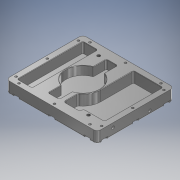
# Autodesk Inventor part: bottom plate mod
Saved by Autodesk Inventor 2017 SP1 (Build 210196100, 196)
## iProperties
Created: 2018-05-03
Part Number: bottom plate mod
Material: Aluminum 6061
Document SubType Name: Modeling
Designer: SimonD
Density: 2.7 g/cm^3
Appearance: Aluminum - Polished
Author: SimonD
Autodesk Inventor part; units mm, degrees
ref_plane "YZ Plane" through (0, 0, 0) normal (1, 0, 0) x (0, 1, 0)
ref_plane "XZ Plane" through (0, 0, 0) normal (0, 1, 0) x (-1, 0, 0)
ref_plane "XY Plane" through (0, 0, 0) normal (0, 0, 1) x (1, 0, 0)
sketch "Sketch1" plane through (0, 0, 0) normal (0, 0, 1) x (1, 0, 0)
  line L0 (-53, 53) -> (53, 53)
  line L1 (53, 53) -> (53, -53)
  line L2 (53, -53) -> (-53, -53)
  line L3 (-53, -53) -> (-53, 53)
  line L4 (-53, 53) -> (53, -53) construction
  line L5 (53, 53) -> (-53, -53) construction
  point P0 (0, 0)
  dimension "d0" = 106
  dimension "d1" = 106
  constraints: 12 end point, 2 midpoint, 2 parallel, 1 horizontal, 1 perpendicular
  measures "d0" distance of L1.end L2.end
  measures "d1" distance between parallel lines of L2 L0
extrude "Extrusion1" add sketch "Sketch1" along normal blind 16
sketch "Sketch3" plane through (0, 0, 16) normal (0, 0, 1) x (1, 0, 0)
  circle A0 centre (0, 0) radius 23.25
  dimension "d21" = 46.5
  constraints: 1 centre point, 1 coincident
  measures "d21" diameter of A0
extrude "Extrusion2" cut sketch "Sketch3" against normal blind 12
thicken "Thicken1" operation add thickness 20 both sides no extend neighbours yes toward (1, 0, 0) faces at (53, 17.6667, 5.3333)
fillet "Fillet3" radius 5 4 edges at (-53, -53, 8) (-53, 53, 8) (73, -53, 8) (73, 53, 8)
sketch "Sketch4" plane through (0, 0, 0) normal (0, 0, -1) x (-1, 0, 0)
  line L0 (48, 53) -> (-68, 53) projected
  line L1 (-73, 48) -> (-73, -48) projected
  line L2 (53, -48) -> (53, 48) projected
  line L3 (-68, -53) -> (48, -53) projected
  point P0 (0, 0)
  point P1 (-59, 49)
  point P2 (-69, 0)
  point P3 (-59, -49)
  point P4 (-10, -49)
  point P5 (39, -49)
  point P6 (49, 0)
  point P7 (39, 49)
  point P8 (-10, 49)
  point P9 (49, 43)
  point P10 (49, -43)
  point P11 (-69, 43)
  point P12 (-69, -43)
  dimension "d28" = 4
  dimension "d29" = 14
  dimension "d30" = 14
  dimension "d31" = 4
  dimension "d32" = 4
  dimension "d33" = 4
  dimension "d34" = 14
  dimension "d35" = 4
  dimension "d36" = 14
  dimension "d37" = 4
  dimension "d38" = 4
  dimension "d39" = 63
  dimension "d40" = 63
  dimension "d43" = 10
  dimension "d44" = 10
  dimension "d45" = 4
  dimension "d53" = 4
  measures "d28" distance from line of point (-59, 49) L0
  measures "d29" distance from line of point (-59, 49) L1
  measures "d30" distance from line of point (39, 49) L2
  measures "d31" distance from line of point (-10, 49) L0
  measures "d32" distance from line of point (-69, 0) L1
  measures "d33" distance from line of point (-59, -49) L3
  measures "d34" distance from line of point (-59, -49) L1
  measures "d35" distance from line of point (39, -49) L3
  measures "d36" distance from line of point (39, -49) L2
  measures "d37" distance from line of point (-10, -49) L3
  measures "d38" distance from line of point (49, 0) L2
  measures "d39" distance from line of point (-10, 49) L1
  measures "d40" distance from line of point (-10, -49) L1
  measures "d43" distance from line of point (49, 43) L0
  measures "d44" distance from line of point (49, -43) L3
  measures "d45" distance from line of point (49, -43) L2
  measures "d53" distance from line of point (39, 49) L0
hole "Hole2" at (59, 49, 0) at (69, 0, 0) at (59, -49, 0) at (10, -49, 0) at (-39, -49, 0) at (-49, 0, 0) at (-39, 49, 0) at (10, 49, 0) at (-49, 43, 0) at (-49, -43, 0) at (69, -43, 0) at (69, 43, 0) direction (0, 0, 1) diameter 3.1 end through all
fillet "Fillet5" radius 2 8 edges at (71.5355, 51.5355, 0) (73, 0, 0) (71.5355, -51.5355, 0) (10, -53, 0) (-51.5355, -51.5355, 0) (-53, 0, 0) (-51.5355, 51.5355, 0) (10, 53, 0)
sketch "Sketch7" plane through (0, 0, 16) normal (0, 0, 1) x (1, 0, 0)
  line L0 (7.5, -40) -> (-7.5, -40)
  line L1 (-7.5, -40) -> (-7.5, 40)
  line L2 (-7.5, 40) -> (7.5, 40)
  line L3 (7.5, 40) -> (7.5, -40)
  line L4 (7.5, -40) -> (-7.5, 40) construction
  line L5 (-7.5, -40) -> (7.5, 40) construction
  point P0 (0, 0)
  dimension "d78" = 15
  dimension "d157" = 40
  constraints: 12 end point, 2 midpoint, 2 parallel, 1 horizontal, 1 perpendicular
  measures "d78" distance of L1.end L2.end
  measures "d157" distance from line of L2 point (0, 0)
extrude "Extrusion4" cut sketch "Sketch7" against normal blind 12
fillet "Fillet6" radius 2 4 edges at (-7.5, 40, 10) (7.5, 40, 10) (-7.5, -40, 10) (7.5, -40, 10)
chamfer "Chamfer1" distance 0.5 angle 45 16 edges at (6.9142, -39.4142, 16) (7.5, -30.0036, 16) (0, -40, 16) (-6.9142, -39.4142, 16) (-7.5, -30.0036, 16) (-23.25, 0, 16) (-7.5, 30.0036, 16) (-6.9142, 39.4142, 16) (0, 40, 16) (6.9142, 39.4142, 16) (7.5, 30.0036, 16) (-7.5, 22.0071, 10) (7.5, 22.0071, 10) (-7.5, -22.0071, 10) (7.5, -22.0071, 10) (23.25, 0, 16)
sketch "Sketch8" plane through (0, 0, 0) normal (0, 0, -1) x (-1, 0, 0)
  circle A0 centre (39, -49) radius 1.55 projected
  circle A1 centre (49, -43) radius 1.55 projected
  circle A2 centre (49, 0) radius 1.55 projected
  circle A3 centre (-59, -49) radius 1.55 projected
  circle A4 centre (-69, 0) radius 1.55 projected
  circle A5 centre (-59, 49) radius 1.55 projected
  circle A6 centre (-10, 49) radius 1.55 projected
  circle A7 centre (39, 49) radius 1.55 projected
  circle A8 centre (49, 43) radius 1.55 projected
  line L0 (53, -3) -> (46, -3)
  line L1 (46, -3) -> (46, 3)
  line L2 (46, 3) -> (53, 3)
  line L3 (53, 3) -> (53, -3)
  line L4 (53, -48) -> (53, 48) projected
  line L5 (53, 40) -> (46, 40)
  line L6 (46, 40) -> (46, 46)
  line L7 (46, 46) -> (53, 46)
  line L8 (53, 46) -> (53, 40)
  line L9 (48, 53) -> (-68, 53) projected
  line L10 (42, 46) -> (36, 46)
  line L11 (36, 46) -> (36, 53)
  line L12 (36, 53) -> (42, 53)
  line L13 (42, 53) -> (42, 46)
  line L14 (-7, 46) -> (-13, 46)
  line L15 (-13, 46) -> (-13, 53)
  line L16 (-13, 53) -> (-7, 53)
  line L17 (-7, 53) -> (-7, 46)
  line L18 (-56, 46) -> (-62, 46)
  line L19 (-62, 46) -> (-62, 53)
  line L20 (-62, 53) -> (-56, 53)
  line L21 (-56, 53) -> (-56, 46)
  line L22 (-73, -3) -> (-66, -3)
  line L23 (-66, -3) -> (-66, 3)
  line L24 (-66, 3) -> (-73, 3)
  line L25 (-73, 3) -> (-73, -3)
  line L26 (-56, -53) -> (-62, -53)
  line L27 (-62, -53) -> (-62, -46)
  line L28 (-62, -46) -> (-56, -46)
  line L29 (-56, -46) -> (-56, -53)
  line L30 (42, -53) -> (36, -53)
  line L31 (36, -53) -> (36, -46)
  line L32 (36, -46) -> (42, -46)
  line L33 (42, -46) -> (42, -53)
  line L34 (53, -46) -> (46, -46)
  line L35 (46, -46) -> (46, -40)
  line L36 (46, -40) -> (53, -40)
  line L37 (53, -40) -> (53, -46)
  line L38 (-7, -53) -> (-13, -53)
  line L39 (-13, -53) -> (-13, -46)
  line L40 (-13, -46) -> (-7, -46)
  line L41 (-7, -46) -> (-7, -53)
  circle A9 centre (-10, -49) radius 1.55 projected
  line L42 (-73, 48) -> (-73, -48) projected
  line L43 (-73, 40) -> (-66, 40)
  line L44 (-66, 40) -> (-66, 46)
  line L45 (-66, 46) -> (-73, 46)
  line L46 (-73, 46) -> (-73, 40)
  line L47 (-73, -46) -> (-66, -46)
  line L48 (-66, -46) -> (-66, -40)
  line L49 (-66, -40) -> (-73, -40)
  line L50 (-73, -40) -> (-73, -46)
  circle A10 centre (-69, -43) radius 1.55 projected
  circle A11 centre (-69, 43) radius 1.55 projected
  point P0 (0, 0)
  point P1 (-7, -53)
  dimension "d85" = 3
  dimension "d86" = 3
  dimension "d87" = 3
  dimension "d88" = 3
  dimension "d89" = 3
  dimension "d90" = 3
  dimension "d91" = 3
  dimension "d92" = 3
  dimension "d93" = 3
  dimension "d94" = 3
  dimension "d95" = 3
  dimension "d96" = 3
  dimension "d97" = 3
  dimension "d98" = 3
  dimension "d99" = 3
  dimension "d102" = 3
  dimension "d103" = 3
  dimension "d107" = 3
  dimension "d108" = 3
  dimension "d109" = 3
  dimension "d143" = 3
  dimension "d144" = 3
  dimension "d145" = 3
  dimension "d146" = 3
  dimension "d147" = 3
  dimension "d148" = 3
  dimension "d149" = 3
  dimension "d150" = 3
  dimension "d151" = 3
  dimension "d190" = 0
  constraints: 96 end point, 24 parallel, 15 point on line, 12 coincident, 12 horizontal, 12 perpendicular
  measures "d85" distance from line of L33 point (39, -49)
  measures "d86" distance from line of L32 point (39, -49)
  measures "d87" distance from line of L31 A0.centre
  measures "d88" distance from line of L36 point (49, -43)
  measures "d89" distance from line of L35 point (49, -43)
  measures "d90" distance from line of L0 point (49, 0)
  measures "d91" distance from line of L2 point (49, 0)
  measures "d92" distance from line of L1 point (49, 0)
  measures "d93" distance from line of point (49, 43) L5
  measures "d94" distance from line of L7 point (49, 43)
  measures "d95" distance from line of L13 point (39, 49)
  measures "d96" distance from line of L17 point (-10, 49)
  measures "d97" distance from line of L15 point (-10, 49)
  measures "d98" distance from line of L21 point (-59, 49)
  measures "d99" distance from line of L19 point (-59, 49)
  measures "d102" distance from line of L23 point (-69, 0)
  measures "d103" distance from line of L24 point (-69, 0)
  measures "d107" distance from line of L29 point (-59, -49)
  measures "d108" distance from line of L27 A3.centre
  measures "d109" distance from line of L28 A3.centre
  measures "d143" distance from line of L41 point (-10, -49)
  measures "d144" distance from line of L39 point (-10, -49)
  measures "d145" distance from line of L40 point (-10, -49)
  measures "d146" distance from line of L43 point (-69, 43)
  measures "d147" distance from line of L45 point (-69, 43)
  measures "d148" distance from line of L44 point (-69, 43)
  measures "d149" distance from line of L47 A10.centre
  measures "d150" distance from line of L49 point (-69, -43)
  measures "d151" distance from line of L48 A10.centre
  measures "d190" distance between parallel lines of L3 L4
sketch "Sketch9" plane through (0, 0, 16) normal (0, 0, 1) x (1, 0, 0)
  line L0 (73, -48) -> (73, 48) projected
  line L1 (-53, 48) -> (-53, -48) projected
  point P0 (0, 0)
  point P1 (69, 25)
  point P2 (69, -25)
  point P3 (-49, 25)
  point P4 (-49, -25)
  dimension "d116" = 25
  dimension "d117" = 4
  dimension "d118" = 25
  dimension "d119" = 4
  dimension "d120" = 4
  dimension "d121" = 4
  measures "d116" vertical distance of point (69, 25) point (0, 0)
  measures "d117" distance from line of point (69, 25) L0
  measures "d118" vertical distance of point (69, -25) point (0, 0)
  measures "d119" distance from line of point (69, -25) L0
  measures "d120" distance from line of point (-49, 25) L1
  measures "d121" distance from line of point (-49, -25) L1
hole "Hole4" [suppressed]
sketch "Sketch10" plane through (0, 0, 16) normal (0, 0, 1) x (1, 0, 0)
  line L0 (25, 45) -> (65, 45)
  line L1 (65, 45) -> (65, -35)
  line L2 (65, -35) -> (25, -35)
  line L3 (25, -35) -> (25, 45)
  line L4 (73, -48) -> (73, 48) projected
  point P0 (0, 0)
  dimension "d129" = 45
  dimension "d130" = 35
  dimension "d131" = 25
  dimension "d132" = 8
  constraints: 8 end point, 2 parallel, 1 horizontal, 1 perpendicular
  measures "d129" distance from line of L0 point (0, 0)
  measures "d130" distance from line of L2 point (0, 0)
  measures "d131" distance from line of L3 point (0, 0)
  measures "d132" distance between parallel lines of L1 L4
extrude "Extrusion6" cut sketch "Sketch10" against normal blind 14.5
fillet "Fillet8" radius 2 4 edges at (25, 45, 8.75) (65, 45, 8.75) (25, -35, 8.75) (65, -35, 8.75)
sketch "Sketch11" plane through (0, 0, 16) normal (0, 0, 1) x (1, 0, 0)
  line L0 (-45, 45) -> (-25, 45)
  line L1 (-25, 45) -> (-25, -45)
  line L2 (-25, -45) -> (-45, -45)
  line L3 (-45, -45) -> (-45, 45)
  line L4 (-53, 48) -> (-53, -48) projected
  point P0 (0, 0)
  dimension "d136" = 45
  dimension "d137" = 45
  dimension "d138" = 8
  dimension "d139" = 20
  constraints: 8 end point, 2 parallel, 1 horizontal, 1 perpendicular
  measures "d136" distance from line of L0 point (0, 0)
  measures "d137" distance from line of L2 point (0, 0)
  measures "d138" distance between parallel lines of L3 L4
  measures "d139" distance between parallel lines of L1 L3
extrude "Extrusion7" cut sketch "Sketch11" against normal blind 14
fillet "Fillet9" radius 2 4 edges at (-25, 45, 9) (-45, 45, 9) (-45, -45, 9) (-25, -45, 9)
extrude "Extrusion8" cut sketch "Sketch8" against normal blind 3.2
fillet "Fillet10" radius 3 24 edges at (-46, -46, 1.6) (-46, -40, 1.6) (-42, -46, 1.6) (-36, -46, 1.6) (-46, -3, 1.6) (-46, 3, 1.6) (-46, 40, 1.6) (-46, 46, 1.6) (-42, 46, 1.6) (-36, 46, 1.6) (7, 46, 1.6) (13, 46, 1.6) (56, 46, 1.6) (62, 46, 1.6) (66, 40, 1.6) (66, 46, 1.6) (66, -3, 1.6) (66, 3, 1.6) (66, -40, 1.6) (66, -46, 1.6) (62, -46, 1.6) (56, -46, 1.6) (13, -46, 1.6) (7, -46, 1.6)
sketch "Sketch12" plane through (0, 0, 16) normal (0, 0, 1) x (1, 0, 0)
  line L0 (30, -35) -> (14, -35)
  line L1 (14, -35) -> (14, -21)
  line L2 (14, -21) -> (30, -21)
  line L3 (30, -21) -> (30, -35)
  line L4 (-48, -53) -> (68, -53) projected
  point P0 (0, 0)
  dimension "d161" = 16
  dimension "d195" = 14
  dimension "d196" = 14
  constraints: 8 end point, 2 parallel, 1 horizontal, 1 perpendicular
  measures "d161" distance of L1.end L2.end
  measures "d195" distance between parallel lines of L2 L0
  measures "d196" distance from line of L1 point (0, 0)
extrude "Extrusion9" cut sketch "Sketch12" against normal blind 14.5
fillet "Fillet11" radius 25 1 edges at (25, -21, 8.75)
sketch "Sketch13" plane through (73, -48, 16) normal (1, 0, 0) x (0, 0, -1)
  line L0 (12, 86) -> (0.5, 86) projected
  line L1 (0, -5) -> (14, -5) projected
  line L2 (16, 0) -> (16, 96) projected
  line L3 (16, 0) -> (16, 96) projected
  point P0 (16, 48)
  point P1 (6, 17)
  point P2 (16, 8)
  point P3 (16, 45)
  point P4 (11, 67.6)
  point P5 (16, 51)
  point P6 (16, 88)
  point P7 (16, -5)
  point P8 (0, 86)
  dimension "d168" = 22
  dimension "d169" = 10
  dimension "d170" = 72.6
  dimension "d171" = 5
  measures "d168" distance from line of point (6, 17) L1
  measures "d169" distance from line of point (6, 17) L2
  measures "d170" distance from line of point (11, 67.6) L1
  measures "d171" distance from line of point (11, 67.6) L3
hole "Hole5" at (73, -31, 10) at (73, 19.6, 5) direction (-1, 0, 0) diameter 2.013 depth 10 tip angle 118 counterbore diameter 4 counterbore depth 3 thread size "M2.5x0.45" class "6H" standard "ISO Metric profile"
sketch "Sketch14" plane through (0, 0, 0) normal (0, 0, -1) x (-1, 0, 0)
  line L0 (48, 53) -> (-68, 53) projected
  line L1 (53, -48) -> (53, 48) projected
  line L2 (-73, 48) -> (-73, -48) projected
  line L3 (-68, -53) -> (48, -53) projected
  point P0 (0, 0)
  point P1 (-47, -39)
  point P2 (17, 39)
  point P3 (36, 53)
  point P4 (-7, 53)
  point P5 (53, -40)
  point P6 (53, 40)
  point P7 (-73, -3)
  point P8 (-73, -40)
  point P9 (-56, -53)
  point P10 (-13, -53)
  dimension "d179" = 14
  dimension "d180" = 36
  dimension "d181" = 26
  dimension "d182" = 14
  measures "d179" distance from line of point (17, 39) L0
  measures "d180" distance from line of point (17, 39) L1
  measures "d181" distance from line of point (-47, -39) L2
  measures "d182" distance from line of point (-47, -39) L3
hole "Hole6" at (47, -39, 0) at (-17, 39, 0) direction (0, 0, 1) diameter 4.134 end through all thread size "M5x0.8" class "6H" standard "ISO Metric profile"
fillet "Fillet13" radius 1.5 24 edges at (-53, 40, 2.6) (-53, 46, 2.6) (-42, 53, 2.6) (-36, 53, 2.6) (7, 53, 2.6) (13, 53, 2.6) (56, 53, 2.6) (62, 53, 2.6) (73, 46, 2.6) (73, 40, 2.6) (73, 3, 2.6) (73, -3, 2.6) (73, -40, 2.6) (73, -46, 2.6) (62, -53, 2.6) (56, -53, 2.6) (7, -53, 2.6) (13, -53, 2.6) (-36, -53, 2.6) (-42, -53, 2.6) (-53, -46, 2.6) (-53, -40, 2.6) (-53, -3, 2.6) (-53, 3, 2.6)
sketch "Sketch15" plane through (0, 0, 16) normal (0, 0, 1) x (1, 0, 0)
  line L0 (63, -35) -> (14, -35) projected
  line L1 (14, -35) -> (36, -35)
  line L2 (36, -35) -> (36, -40)
  line L3 (36, -40) -> (14, -40)
  line L4 (14, -40) -> (14, -35)
  line L5 (14, -35) -> (14, -21) projected
  point P0 (0, 0)
  point P1 (12, -20.4954)
  dimension "d197" = 5
  dimension "d198" = 22
  constraints: 8 end point, 2 parallel, 1 horizontal, 1 perpendicular, 1 other
  measures "d197" distance between parallel lines of L3 L0
extrude "Extrusion10" cut sketch "Sketch15" against normal blind 14.5
fillet "Fillet14" radius 3 4 edges at (14, -40, 8.75) (14, -21, 8.75) (36, -40, 8.75) (36, -35, 8.75)
chamfer "Chamfer4" distance 0.5 angle 45 22 edges at (25, -40, 16) (14.8787, -39.1213, 16) (14, -29.7681, 16) (14.3107, -21.2067, 16) (22.4105, -11.3678, 16) (25, 21.3562, 16) (25.5858, 44.4142, 16) (45, 45, 16) (64.4142, 44.4142, 16) (65, 5, 16) (64.4142, -34.4142, 16) (50.958, -35, 16) (36.9796, -35.7087, 16) (34.9365, -39.2913, 16) (-35, -45, 16) (-44.4142, -44.4142, 16) (-45, 0, 16) (-44.4142, 44.4142, 16) (-35, 45, 16) (-25.5858, 44.4142, 16) (-25, 0, 16) (-25.5858, -44.4142, 16)
body "Solid1"
